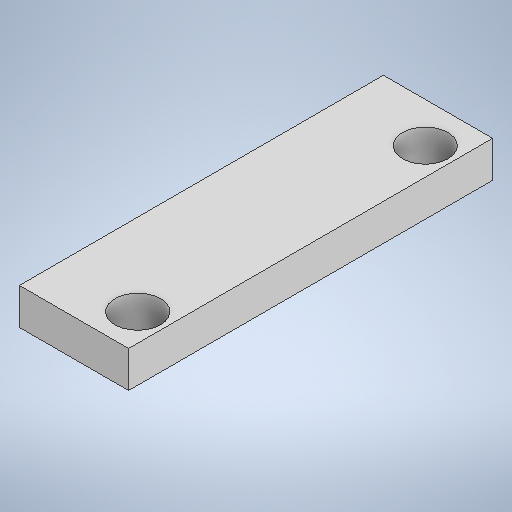
# Autodesk Inventor part: B1 fermeture
Saved by Autodesk Inventor 2025 (Build 290162000, 162)
## iProperties
Created: 2025-01-19
Part Number: B1 fermeture
Material: Generic
Document SubType Name: Modeling
Designer: Pauline Simonnet
Density: 1 g/cm^3
Appearance: Default
Author: Pauline Simonnet
Autodesk Inventor part; units mm, degrees
ref_plane "YZ Plane" through (0, 0, 0) normal (1, 0, 0) x (0, 1, 0)
ref_plane "XZ Plane" through (0, 0, 0) normal (0, 1, 0) x (-1, 0, 0)
ref_plane "XY Plane" through (0, 0, 0) normal (0, 0, 1) x (1, 0, 0)
sketch "Sketch1" plane through (0, 0, 0) normal (0, 1, 0) x (-1, 0, 0)
  line L0 (0, 0) -> (12, 0)
  line L1 (12, 0) -> (12, -40)
  line L2 (12, -40) -> (0, -40)
  line L3 (0, -40) -> (0, 0)
  dimension "d0" = 40
  dimension "d1" = 12
  constraints: 8 end point, 2 parallel, 1 horizontal, 1 perpendicular
  measures "d0" distance between parallel lines of L2 L0
  measures "d1" distance of L1.end L2.end
extrude "Extrusion1" add sketch "Sketch1" along normal blind 4
sketch "Sketch2" plane through (0, 4, 0) normal (0, 1, 0) x (1, 0, 0)
  circle A0 centre (-3, 4) radius 2.5
  circle A1 centre (-3, 35.6) radius 2.5
  line L0 (-12, 0) -> (0, 0) projected
  line L1 (0, 0) -> (0, 40) projected
  dimension "d4" = 5
  dimension "d5" = 5
  dimension "d6" = 4
  dimension "d7" = 3
  dimension "d8" = 31.6
  dimension "d9" = 3
  constraints: 2 centre point
  measures "d4" diameter of A0
  measures "d5" diameter of A1
  measures "d6" distance from line of A0.centre L0
  measures "d7" distance from line of L1 A0.centre
  measures "d8" distance of A1.centre A0.centre
  measures "d9" distance from line of L1 A1.centre
extrude "Extrusion2" cut sketch "Sketch2" against normal blind 4
sketch "Sketch3" plane through (0, 0, 0) normal (0, -1, 0) x (1, 0, 0)
  line L0 (-12, -30) -> (-6, -30)
  line L1 (-6, -30) -> (-6, -10)
  line L2 (-6, -10) -> (-12, -10)
  line L3 (-12, -10) -> (-12, -30)
  line L4 (0, -40) -> (-12, -40) projected
  line L5 (-12, 0) -> (0, 0) projected
  line L6 (-12, -40) -> (-12, 0) projected
  dimension "d12" = 6
  dimension "d15" = 10
  dimension "d16" = 10
  dimension "d17" = 0
  constraints: 8 end point, 2 parallel, 1 horizontal, 1 perpendicular
  measures "d12" distance between parallel lines of L3 L1
  measures "d15" distance between parallel lines of L0 L4
  measures "d16" distance between parallel lines of L5 L2
  measures "d17" distance between parallel lines of L6 L3
extrude "Extrusion3" add sketch "Sketch3" along normal blind 4.4
equation "\"d5\" = d4"
equation "\"d9\" = d7"
body "Solid1"
